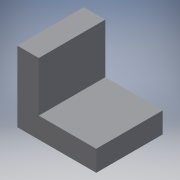
# Autodesk Inventor part: FilletsChamfers
Saved by Autodesk Inventor 2018 (Build 220112000, 112)
## iProperties
Created: 2005-07-15
Part Number: FilletsChamfers
Document SubType Name: Modeling
Designer: Administrator
Manufacturer: Standard
Standards Organization: Custom
Material: Generic
Density: 1 g/cm^3
Appearance: Default
Author: Administrator
Autodesk Inventor part; units mm, degrees
ref_plane "YZ Plane" through (0, 0, 0) normal (1, 0, 0) x (0, 1, 0)
ref_plane "XZ Plane" through (0, 0, 0) normal (0, 1, 0) x (-1, 0, 0)
ref_plane "XY Plane" through (0, 0, 0) normal (0, 0, 1) x (1, 0, 0)
sketch "Sketch1" plane through (0, 0, 0) normal (0, 0, 1) x (1, 0, 0)
  line L0 (-34.925, -3.175) -> (25.4, -3.175)
  line L1 (25.4, -3.175) -> (25.4, -19.05)
  line L2 (25.4, -19.05) -> (-34.925, -19.05)
  line L3 (-34.925, -19.05) -> (-34.925, -3.175)
  line L4 (-34.925, -19.05) -> (-18.4918, -19.05)
  line L5 (-18.4918, -19.05) -> (-18.4918, 34.925)
  line L6 (-18.4918, 34.925) -> (-34.925, 34.925)
  line L7 (-34.925, 34.925) -> (-34.925, -19.05)
  constraints: 16 end point, 4 parallel, 2 horizontal, 2 perpendicular
extrude "Extrusion1" add sketch "Sketch1" along normal blind 50.8
shell "Shell1" thickness 2.54 removed faces 1 at (-14.8167, -19.05, 16.9333)
fillet "Fillet2" radius 3.175 8 edges at (-32.385, -19.05, 25.4) (-4.7625, -19.05, 2.54) (-21.0318, -5.715, 25.4) (22.86, -5.715, 25.4) (22.86, -19.05, 25.4) (-4.7625, -19.05, 48.26) (-32.385, 32.385, 25.4) (-21.0318, 32.385, 25.4)
body "Solid1"
